Autodesk Inventor part; units mm, degrees
(part 3 of 3)
sketch "스케치33" plane through (0, 0, 2) normal (0, 0, 1) x (1, 0, 0)
  circle A0 centre (-11.9, -60) radius 1.35 projected
  line L0 (-6.96, -60.06) -> (-6.96, -57.94) projected
  arc A1 (-4.76, -57.94) -> (-6.96, -57.94) centre (-5.86, -57.94) ccw projected
  line L1 (-4.76, -57.94) -> (4.96, -57.94) projected
  arc A2 (7.16, -57.94) -> (4.96, -57.94) centre (6.06, -57.94) ccw projected
  line L2 (7.16, -57.94) -> (7.16, -60.06) projected
  arc A3 (4.96, -60.06) -> (7.16, -60.06) centre (6.06, -60.06) ccw projected
  line L3 (4.96, -60.06) -> (-4.76, -60.06) projected
  arc A4 (-6.96, -60.06) -> (-4.76, -60.06) centre (-5.86, -60.06) ccw projected
  circle A5 centre (12.1, -60) radius 1.35 projected
  line L4 (-14.9, -62) -> (15.1, -62) projected
  line L5 (15.1, -62) -> (15.1, -54.5339) projected
  arc A6 (15.1, -54.5339) -> (14.9713, -53.4701) centre (10.639, -54.5339) ccw projected
  line L6 (14.9713, -53.4701) -> (6.3746, -18.4593) projected
  arc A7 (6.3746, -18.4593) -> (-6.1746, -18.4593) centre (0.1, -20) ccw projected
  line L7 (-6.1746, -18.4593) -> (-14.7713, -53.4701) projected
  arc A8 (-14.7713, -53.4701) -> (-14.9, -54.5339) centre (-10.439, -54.5339) ccw projected
  line L8 (-14.9, -54.5339) -> (-14.9, -62) projected
  line L9 (-8.6217, -47.1327) -> (-4.5428, -30.5211) projected
  arc A9 (-0.3945, -27.4837) -> (-4.5428, -30.5211) centre (-0.6582, -31.475) ccw projected
  arc A10 (-0.3945, -27.4837) -> (0.5945, -27.4837) centre (0.1, -20) ccw projected
  arc A11 (4.7428, -30.5211) -> (0.5945, -27.4837) centre (0.8582, -31.475) ccw projected
  line L10 (4.7428, -30.5211) -> (8.8217, -47.1327) projected
  arc A12 (5.616, -52.0285) -> (8.8217, -47.1327) centre (4.9371, -48.0865) ccw projected
  arc A13 (-5.416, -52.0285) -> (5.616, -52.0285) centre (0.1, -20) ccw projected
  arc A14 (-8.6217, -47.1327) -> (-5.416, -52.0285) centre (-4.7371, -48.0865) ccw projected
  circle A15 centre (0.1, -20) radius 4 projected
  circle A16 centre (0.1, -20) radius 4 projected
  line L11 (-15.822, -62) -> (16.178, -62) projected
  line L12 (16.178, -62) -> (16.178, -54.5339) projected
  arc A17 (16.178, -54.5339) -> (16.0205, -53.2317) centre (10.717, -54.5339) ccw projected
  line L13 (16.0205, -53.2317) -> (7.4238, -18.2208) projected
  arc A18 (7.4238, -18.2208) -> (-7.0677, -18.2208) centre (0.178, -20) ccw projected
  line L14 (-7.0677, -18.2208) -> (-15.6644, -53.2317) projected
  arc A19 (-15.6644, -53.2317) -> (-15.822, -54.5339) centre (-10.361, -54.5339) ccw projected
  line L15 (-15.822, -54.5339) -> (-15.822, -62) projected
  circle A20 centre (11.1, -45.3) radius 1.35 projected
  line L16 (8.16, -44.34) -> (8.16, -46.26) projected
  arc A21 (7.06, -47.36) -> (8.16, -46.26) centre (8.16, -47.36) ccw projected
  line L17 (7.06, -47.36) -> (-6.86, -47.36) projected
  arc A22 (-7.96, -46.26) -> (-6.86, -47.36) centre (-7.96, -47.36) ccw projected
  line L18 (-7.96, -46.26) -> (-7.96, -44.34) projected
  arc A23 (-6.86, -43.24) -> (-7.96, -44.34) centre (-7.96, -43.24) ccw projected
  line L19 (-6.86, -43.24) -> (7.06, -43.24) projected
  arc A24 (8.16, -44.34) -> (7.06, -43.24) centre (8.16, -43.24) ccw projected
  circle A25 centre (-10.9, -45.3) radius 1.35 projected
  arc A26 (-4.9649, -40.6273) -> (5.1649, -40.6273) centre (0.1, -20) ccw projected
  arc A27 (-6.4303, -38.208) -> (-4.9649, -40.6273) centre (-4.488, -38.685) ccw projected
  line L20 (-6.4303, -38.208) -> (-4.5428, -30.5211) projected
  arc A28 (-0.3945, -27.4837) -> (-4.5428, -30.5211) centre (-0.6582, -31.475) ccw projected
  arc A29 (-0.3945, -27.4837) -> (0.5945, -27.4837) centre (0.1, -20) ccw projected
  arc A30 (4.7428, -30.5211) -> (0.5945, -27.4837) centre (0.8582, -31.475) ccw projected
  line L21 (4.7428, -30.5211) -> (6.6303, -38.208) projected
  arc A31 (5.1649, -40.6273) -> (6.6303, -38.208) centre (4.688, -38.685) ccw projected
  point P0 (0, 0)
extrude "돌출33" cut sketch "스케치33" against normal blind 2 contours A0 | L0 A1 L1 A2 L2 A3 L3 A4 | A5
sketch "스케치34" plane through (0, 0, 2) normal (0, 0, 1) x (1, 0, 0)
  circle A0 centre (12.1, -60) radius 1.35 projected
  circle A1 centre (-11.9, -60) radius 1.35 projected
  arc A2 (7.16, -57.94) -> (4.96, -57.94) centre (6.06, -57.94) ccw projected
  line L0 (7.16, -57.94) -> (7.16, -60.06) projected
  arc A3 (4.96, -60.06) -> (7.16, -60.06) centre (6.06, -60.06) ccw projected
  line L1 (4.96, -60.06) -> (-4.76, -60.06) projected
  arc A4 (-6.96, -60.06) -> (-4.76, -60.06) centre (-5.86, -60.06) ccw projected
  line L2 (-6.96, -60.06) -> (-6.96, -57.94) projected
  arc A5 (-4.76, -57.94) -> (-6.96, -57.94) centre (-5.86, -57.94) ccw projected
  line L3 (-4.76, -57.94) -> (4.96, -57.94) projected
  circle A6 centre (0.1, -20) radius 4 projected
  line L4 (-15.822, -62) -> (16.178, -62) projected
  line L5 (16.178, -62) -> (16.178, -54.5339) projected
  arc A7 (16.178, -54.5339) -> (16.0205, -53.2317) centre (10.717, -54.5339) ccw projected
  line L6 (16.0205, -53.2317) -> (7.4238, -18.2208) projected
  arc A8 (7.4238, -18.2208) -> (-7.0677, -18.2208) centre (0.178, -20) ccw projected
  line L7 (-7.0677, -18.2208) -> (-15.6644, -53.2317) projected
  arc A9 (-15.6644, -53.2317) -> (-15.822, -54.5339) centre (-10.361, -54.5339) ccw projected
  line L8 (-15.822, -54.5339) -> (-15.822, -62) projected
  circle A10 centre (11.1, -45.3) radius 1.35 projected
  line L9 (8.16, -44.34) -> (8.16, -46.26) projected
  arc A11 (7.06, -47.36) -> (8.16, -46.26) centre (8.16, -47.36) ccw projected
  line L10 (7.06, -47.36) -> (-6.86, -47.36) projected
  arc A12 (-7.96, -46.26) -> (-6.86, -47.36) centre (-7.96, -47.36) ccw projected
  line L11 (-7.96, -46.26) -> (-7.96, -44.34) projected
  arc A13 (-6.86, -43.24) -> (-7.96, -44.34) centre (-7.96, -43.24) ccw projected
  line L12 (-6.86, -43.24) -> (7.06, -43.24) projected
  arc A14 (8.16, -44.34) -> (7.06, -43.24) centre (8.16, -43.24) ccw projected
  circle A15 centre (-10.9, -45.3) radius 1.35 projected
  arc A16 (-4.9649, -40.6273) -> (5.1649, -40.6273) centre (0.1, -20) ccw projected
  arc A17 (-6.4303, -38.208) -> (-4.9649, -40.6273) centre (-4.488, -38.685) ccw projected
  line L13 (-6.4303, -38.208) -> (-4.5428, -30.5211) projected
  arc A18 (-0.3945, -27.4837) -> (-4.5428, -30.5211) centre (-0.6582, -31.475) ccw projected
  arc A19 (-0.3945, -27.4837) -> (0.5945, -27.4837) centre (0.1, -20) ccw projected
  arc A20 (4.7428, -30.5211) -> (0.5945, -27.4837) centre (0.8582, -31.475) ccw projected
  line L14 (4.7428, -30.5211) -> (6.6303, -38.208) projected
  arc A21 (5.1649, -40.6273) -> (6.6303, -38.208) centre (4.688, -38.685) ccw projected
  circle A22 centre (-11.9, -60) radius 1.35 projected
  line L15 (-6.96, -60.06) -> (-6.96, -57.94) projected
  arc A23 (-4.76, -57.94) -> (-6.96, -57.94) centre (-5.86, -57.94) ccw projected
  line L16 (-4.76, -57.94) -> (4.96, -57.94) projected
  arc A24 (7.16, -57.94) -> (4.96, -57.94) centre (6.06, -57.94) ccw projected
  line L17 (7.16, -57.94) -> (7.16, -60.06) projected
  arc A25 (4.96, -60.06) -> (7.16, -60.06) centre (6.06, -60.06) ccw projected
  line L18 (4.96, -60.06) -> (-4.76, -60.06) projected
  arc A26 (-6.96, -60.06) -> (-4.76, -60.06) centre (-5.86, -60.06) ccw projected
  circle A27 centre (12.1, -60) radius 1.35 projected
  line L19 (-14.9, -62) -> (15.1, -62) projected
  line L20 (15.1, -62) -> (15.1, -54.5339) projected
  arc A28 (15.1, -54.5339) -> (14.9713, -53.4701) centre (10.639, -54.5339) ccw projected
  line L21 (14.9713, -53.4701) -> (6.3746, -18.4593) projected
  arc A29 (6.3746, -18.4593) -> (-6.1746, -18.4593) centre (0.1, -20) ccw projected
  line L22 (-6.1746, -18.4593) -> (-14.7713, -53.4701) projected
  arc A30 (-14.7713, -53.4701) -> (-14.9, -54.5339) centre (-10.439, -54.5339) ccw projected
  line L23 (-14.9, -54.5339) -> (-14.9, -62) projected
  line L24 (-8.6217, -47.1327) -> (-4.5428, -30.5211) projected
  arc A31 (-0.3945, -27.4837) -> (-4.5428, -30.5211) centre (-0.6582, -31.475) ccw projected
  arc A32 (-0.3945, -27.4837) -> (0.5945, -27.4837) centre (0.1, -20) ccw projected
  arc A33 (4.7428, -30.5211) -> (0.5945, -27.4837) centre (0.8582, -31.475) ccw projected
  line L25 (4.7428, -30.5211) -> (8.8217, -47.1327) projected
  arc A34 (5.616, -52.0285) -> (8.8217, -47.1327) centre (4.9371, -48.0865) ccw projected
  arc A35 (-5.416, -52.0285) -> (5.616, -52.0285) centre (0.1, -20) ccw projected
  arc A36 (-8.6217, -47.1327) -> (-5.416, -52.0285) centre (-4.7371, -48.0865) ccw projected
  circle A37 centre (0.1, -20) radius 4 projected
  point P0 (0, 0)
extrude "돌출34" cut sketch "스케치34" against normal blind 2 contours L8 A9 L7 A8 L6 A7 L5 L4 L20 A28 L21 A29 L22 A30 L23
sketch "스케치35" plane through (0, 0, 2) normal (0, 0, 1) x (1, 0, 0)
  arc A0 (-4.9649, -40.6273) -> (5.1649, -40.6273) centre (0.1, -20) ccw projected
  arc A1 (-6.4303, -38.208) -> (-4.9649, -40.6273) centre (-4.488, -38.685) ccw projected
  line L0 (-6.4303, -38.208) -> (-4.5428, -30.5211) projected
  arc A2 (-0.3945, -27.4837) -> (-4.5428, -30.5211) centre (-0.6582, -31.475) ccw projected
  arc A3 (-0.3945, -27.4837) -> (0.5945, -27.4837) centre (0.1, -20) ccw projected
  arc A4 (4.7428, -30.5211) -> (0.5945, -27.4837) centre (0.8582, -31.475) ccw projected
  line L1 (4.7428, -30.5211) -> (6.6303, -38.208) projected
  arc A5 (5.1649, -40.6273) -> (6.6303, -38.208) centre (4.688, -38.685) ccw projected
  circle A6 centre (-10.9, -45.3) radius 1.35 projected
  line L2 (8.16, -44.34) -> (8.16, -46.26) projected
  arc A7 (7.06, -47.36) -> (8.16, -46.26) centre (8.16, -47.36) ccw projected
  line L3 (7.06, -47.36) -> (-6.86, -47.36) projected
  arc A8 (-7.96, -46.26) -> (-6.86, -47.36) centre (-7.96, -47.36) ccw projected
  line L4 (-7.96, -46.26) -> (-7.96, -44.34) projected
  arc A9 (-6.86, -43.24) -> (-7.96, -44.34) centre (-7.96, -43.24) ccw projected
  line L5 (-6.86, -43.24) -> (7.06, -43.24) projected
  arc A10 (8.16, -44.34) -> (7.06, -43.24) centre (8.16, -43.24) ccw projected
  circle A11 centre (11.1, -45.3) radius 1.35 projected
  line L6 (15.1, -62) -> (15.1, -54.5339) projected
  arc A12 (15.1, -54.5339) -> (14.9713, -53.4701) centre (10.639, -54.5339) ccw projected
  line L7 (14.9713, -53.4701) -> (6.3746, -18.4593) projected
  arc A13 (6.3746, -18.4593) -> (-6.1746, -18.4593) centre (0.1, -20) ccw projected
  line L8 (-6.1746, -18.4593) -> (-14.7713, -53.4701) projected
  arc A14 (-14.7713, -53.4701) -> (-14.9, -54.5339) centre (-10.439, -54.5339) ccw projected
  line L9 (-14.9, -54.5339) -> (-14.9, -62) projected
  line L10 (-14.9, -62) -> (15.1, -62) projected
  circle A15 centre (0.1, -20) radius 4 projected
  arc A16 (7.16, -57.94) -> (4.96, -57.94) centre (6.06, -57.94) ccw projected
  line L11 (7.16, -57.94) -> (7.16, -60.06) projected
  arc A17 (4.96, -60.06) -> (7.16, -60.06) centre (6.06, -60.06) ccw projected
  line L12 (4.96, -60.06) -> (-4.76, -60.06) projected
  arc A18 (-6.96, -60.06) -> (-4.76, -60.06) centre (-5.86, -60.06) ccw projected
  line L13 (-6.96, -60.06) -> (-6.96, -57.94) projected
  arc A19 (-4.76, -57.94) -> (-6.96, -57.94) centre (-5.86, -57.94) ccw projected
  line L14 (-4.76, -57.94) -> (4.96, -57.94) projected
  circle A20 centre (-11.9, -60) radius 1.35 projected
  circle A21 centre (12.1, -60) radius 1.35 projected
  line L15 (16.1, -54.5339) -> (16.1, -63)
  line L16 (16.1, -63) -> (-15.9, -63)
  line L17 (-15.9, -63) -> (-15.9, -54.5339)
  arc A22 (-15.7425, -53.2317) -> (-15.9, -54.5339) centre (-10.439, -54.5339) ccw
  line L18 (-15.7425, -53.2317) -> (-7.1458, -18.2208)
  arc A23 (7.3458, -18.2208) -> (-7.1458, -18.2208) centre (0.1, -20) ccw
  line L19 (7.3458, -18.2208) -> (15.9425, -53.2317)
  arc A24 (16.1, -54.5339) -> (15.9425, -53.2317) centre (10.639, -54.5339) ccw
  line L20 (16.1, -63) -> (-15.9, -63)
  line L21 (-15.9, -63) -> (-15.9, -62)
  line L22 (-15.9, -62) -> (16.1, -62)
  line L23 (16.1, -62) -> (16.1, -63)
  point P0 (0, 0)
  dimension "d134" = 1
  constraints: 18 end point, 6 point on circle, 3 centre point, 2 parallel, 1 horizontal, 1 perpendicular, 7 other
  measures "d134" distance between parallel lines of L6 L15
extrude "돌출35" add sketch "스케치35" against normal blind 2 contours L6 A12 L7 A13 L8 A14 L9 L22 L17 A22 L18 A23 L19 A24 L15
sketch "스케치36" plane through (0, 0, 0) normal (0, 0, -1) x (-1, 0, 0)
  line L0 (-16.1, -62) -> (15.9, -62) projected
  line L1 (15.9, -62) -> (15.9, -54.5339) projected
  arc A0 (15.9, -54.5339) -> (15.7425, -53.2317) centre (10.439, -54.5339) ccw projected
  line L2 (15.7425, -53.2317) -> (7.1458, -18.2208) projected
  arc A1 (7.1458, -18.2208) -> (-7.3458, -18.2208) centre (-0.1, -20) ccw projected
  line L3 (-7.3458, -18.2208) -> (-15.9425, -53.2317) projected
  arc A2 (-15.9425, -53.2317) -> (-16.1, -54.5339) centre (-10.639, -54.5339) ccw projected
  line L4 (-16.1, -54.5339) -> (-16.1, -62) projected
  circle A3 centre (-12.1, -60) radius 1.35 projected
  circle A4 centre (11.9, -60) radius 1.35 projected
  arc A5 (-4.96, -57.94) -> (-7.16, -57.94) centre (-6.06, -57.94) ccw projected
  line L5 (-4.96, -57.94) -> (4.76, -57.94) projected
  arc A6 (6.96, -57.94) -> (4.76, -57.94) centre (5.86, -57.94) ccw projected
  line L6 (6.96, -57.94) -> (6.96, -60.06) projected
  arc A7 (4.76, -60.06) -> (6.96, -60.06) centre (5.86, -60.06) ccw projected
  line L7 (4.76, -60.06) -> (-4.96, -60.06) projected
  arc A8 (-7.16, -60.06) -> (-4.96, -60.06) centre (-6.06, -60.06) ccw projected
  line L8 (-7.16, -60.06) -> (-7.16, -57.94) projected
  arc A9 (-5.1649, -40.6273) -> (4.9649, -40.6273) centre (-0.1, -20) ccw projected
  arc A10 (-6.6303, -38.208) -> (-5.1649, -40.6273) centre (-4.688, -38.685) ccw projected
  line L9 (-6.6303, -38.208) -> (-4.7428, -30.5211) projected
  arc A11 (-0.5945, -27.4837) -> (-4.7428, -30.5211) centre (-0.8582, -31.475) ccw projected
  arc A12 (-0.5945, -27.4837) -> (0.3945, -27.4837) centre (-0.1, -20) ccw projected
  arc A13 (4.5428, -30.5211) -> (0.3945, -27.4837) centre (0.6582, -31.475) ccw projected
  line L10 (4.5428, -30.5211) -> (6.4303, -38.208) projected
  arc A14 (4.9649, -40.6273) -> (6.4303, -38.208) centre (4.488, -38.685) ccw projected
  circle A15 centre (10.9, -45.3) radius 1.35 projected
  line L11 (-8.16, -46.26) -> (-8.16, -44.34) projected
  arc A16 (-7.06, -43.24) -> (-8.16, -44.34) centre (-8.16, -43.24) ccw projected
  line L12 (-7.06, -43.24) -> (6.86, -43.24) projected
  arc A17 (7.96, -44.34) -> (6.86, -43.24) centre (7.96, -43.24) ccw projected
  line L13 (7.96, -44.34) -> (7.96, -46.26) projected
  arc A18 (6.86, -47.36) -> (7.96, -46.26) centre (7.96, -47.36) ccw projected
  line L14 (6.86, -47.36) -> (-7.06, -47.36) projected
  arc A19 (-8.16, -46.26) -> (-7.06, -47.36) centre (-8.16, -47.36) ccw projected
  circle A20 centre (-11.1, -45.3) radius 1.35 projected
  circle A21 centre (-0.1, -20) radius 4 projected
  point P0 (0, 0)
extrude "돌출36" add sketch "스케치36" against normal blind 2 contours L5 A6 L6 A7 L7 A8 L8 A5
sketch "스케치37" plane through (0, 0, 2) normal (0, 0, 1) x (1, 0, 0)
  arc A0 (-5.86, -57.94) -> (-6.96, -59.04) centre (-6.96, -57.94) ccw projected
  line L0 (-5.86, -57.94) -> (6.06, -57.94) projected
  arc A1 (7.16, -59.04) -> (6.06, -57.94) centre (7.16, -57.94) ccw projected
  line L1 (7.16, -59.04) -> (7.16, -62) projected
  line L2 (7.16, -62) -> (15.1, -62) projected
  line L3 (15.1, -62) -> (15.1, -54.5339) projected
  arc A2 (15.1, -54.5339) -> (14.9713, -53.4701) centre (10.639, -54.5339) ccw projected
  line L4 (14.9713, -53.4701) -> (6.3746, -18.4593) projected
  arc A3 (6.3746, -18.4593) -> (-6.1746, -18.4593) centre (0.1, -20) ccw projected
  line L5 (-6.1746, -18.4593) -> (-14.7713, -53.4701) projected
  arc A4 (-14.7713, -53.4701) -> (-14.9, -54.5339) centre (-10.439, -54.5339) ccw projected
  line L6 (-14.9, -54.5339) -> (-14.9, -62) projected
  line L7 (-14.9, -62) -> (-6.96, -62) projected
  line L8 (-6.96, -62) -> (-6.96, -59.04) projected
  circle A5 centre (-11.9, -60) radius 1.35 projected
  circle A6 centre (12.1, -60) radius 1.35 projected
  line L9 (-8.6217, -47.1327) -> (-4.5428, -30.5211) projected
  arc A7 (-0.3945, -27.4837) -> (-4.5428, -30.5211) centre (-0.6582, -31.475) ccw projected
  arc A8 (-0.3945, -27.4837) -> (0.5945, -27.4837) centre (0.1, -20) ccw projected
  arc A9 (4.7428, -30.5211) -> (0.5945, -27.4837) centre (0.8582, -31.475) ccw projected
  line L10 (4.7428, -30.5211) -> (8.8217, -47.1327) projected
  arc A10 (5.616, -52.0285) -> (8.8217, -47.1327) centre (4.9371, -48.0865) ccw projected
  arc A11 (-5.416, -52.0285) -> (5.616, -52.0285) centre (0.1, -20) ccw projected
  arc A12 (-8.6217, -47.1327) -> (-5.416, -52.0285) centre (-4.7371, -48.0865) ccw projected
  circle A13 centre (0.1, -20) radius 4 projected
  arc A14 (-4.9649, -40.6273) -> (5.1649, -40.6273) centre (0.1, -20) ccw projected
  arc A15 (-6.4303, -38.208) -> (-4.9649, -40.6273) centre (-4.488, -38.685) ccw projected
  line L11 (-6.4303, -38.208) -> (-4.5428, -30.5211) projected
  arc A16 (-0.3945, -27.4837) -> (-4.5428, -30.5211) centre (-0.6582, -31.475) ccw projected
  arc A17 (-0.3945, -27.4837) -> (0.5945, -27.4837) centre (0.1, -20) ccw projected
  arc A18 (4.7428, -30.5211) -> (0.5945, -27.4837) centre (0.8582, -31.475) ccw projected
  line L12 (4.7428, -30.5211) -> (6.6303, -38.208) projected
  arc A19 (5.1649, -40.6273) -> (6.6303, -38.208) centre (4.688, -38.685) ccw projected
  circle A20 centre (-10.9, -45.3) radius 1.35 projected
  line L13 (8.16, -44.34) -> (8.16, -46.26) projected
  arc A21 (7.06, -47.36) -> (8.16, -46.26) centre (8.16, -47.36) ccw projected
  line L14 (7.06, -47.36) -> (-6.86, -47.36) projected
  arc A22 (-7.96, -46.26) -> (-6.86, -47.36) centre (-7.96, -47.36) ccw projected
  line L15 (-7.96, -46.26) -> (-7.96, -44.34) projected
  arc A23 (-6.86, -43.24) -> (-7.96, -44.34) centre (-7.96, -43.24) ccw projected
  line L16 (-6.86, -43.24) -> (7.06, -43.24) projected
  arc A24 (8.16, -44.34) -> (7.06, -43.24) centre (8.16, -43.24) ccw projected
  circle A25 centre (11.1, -45.3) radius 1.35 projected
  line L17 (-15.9, -62) -> (16.1, -62) projected
  line L18 (16.1, -62) -> (16.1, -54.5339) projected
  arc A26 (16.1, -54.5339) -> (15.9425, -53.2317) centre (10.639, -54.5339) ccw projected
  line L19 (15.9425, -53.2317) -> (7.3458, -18.2208) projected
  arc A27 (7.3458, -18.2208) -> (-7.1458, -18.2208) centre (0.1, -20) ccw projected
  line L20 (-7.1458, -18.2208) -> (-15.7425, -53.2317) projected
  arc A28 (-15.7425, -53.2317) -> (-15.9, -54.5339) centre (-10.439, -54.5339) ccw projected
  line L21 (-15.9, -54.5339) -> (-15.9, -62) projected
  circle A29 centre (0.1, -20) radius 4 projected
  circle A30 centre (-11.9, -60) radius 1.35 projected
  circle A31 centre (12.1, -60) radius 1.35 projected
  point P0 (0, 0)
extrude "돌출37" cut sketch "스케치37" against normal through all contours L0 A1 L1 L17 L8 A0
sketch "스케치38" plane through (0, 0, 2) normal (0, 0, 1) x (1, 0, 0)
  circle A0 centre (12.1, -60) radius 1.35 projected
  circle A1 centre (-11.9, -60) radius 1.35 projected
  circle A2 centre (0.1, -20) radius 4 projected
  line L0 (-6.96, -62) -> (-6.96, -59.04) projected
  arc A3 (-5.86, -57.94) -> (-6.96, -59.04) centre (-6.96, -57.94) ccw projected
  line L1 (-5.86, -57.94) -> (6.06, -57.94) projected
  arc A4 (7.16, -59.04) -> (6.06, -57.94) centre (7.16, -57.94) ccw projected
  line L2 (7.16, -59.04) -> (7.16, -62) projected
  line L3 (7.16, -62) -> (16.1, -62) projected
  line L4 (16.1, -62) -> (16.1, -54.5339) projected
  arc A5 (16.1, -54.5339) -> (15.9425, -53.2317) centre (10.639, -54.5339) ccw projected
  line L5 (15.9425, -53.2317) -> (7.3458, -18.2208) projected
  arc A6 (7.3458, -18.2208) -> (-7.1458, -18.2208) centre (0.1, -20) ccw projected
  line L6 (-7.1458, -18.2208) -> (-15.7425, -53.2317) projected
  arc A7 (-15.7425, -53.2317) -> (-15.9, -54.5339) centre (-10.439, -54.5339) ccw projected
  line L7 (-15.9, -54.5339) -> (-15.9, -62) projected
  line L8 (-15.9, -62) -> (-6.96, -62) projected
  circle A8 centre (11.1, -45.3) radius 1.35 projected
  line L9 (8.16, -44.34) -> (8.16, -46.26) projected
  arc A9 (7.06, -47.36) -> (8.16, -46.26) centre (8.16, -47.36) ccw projected
  line L10 (7.06, -47.36) -> (-6.86, -47.36) projected
  arc A10 (-7.96, -46.26) -> (-6.86, -47.36) centre (-7.96, -47.36) ccw projected
  line L11 (-7.96, -46.26) -> (-7.96, -44.34) projected
  arc A11 (-6.86, -43.24) -> (-7.96, -44.34) centre (-7.96, -43.24) ccw projected
  line L12 (-6.86, -43.24) -> (7.06, -43.24) projected
  arc A12 (8.16, -44.34) -> (7.06, -43.24) centre (8.16, -43.24) ccw projected
  circle A13 centre (-10.9, -45.3) radius 1.35 projected
  arc A14 (-4.9649, -40.6273) -> (5.1649, -40.6273) centre (0.1, -20) ccw projected
  arc A15 (-6.4303, -38.208) -> (-4.9649, -40.6273) centre (-4.488, -38.685) ccw projected
  line L13 (-6.4303, -38.208) -> (-4.5428, -30.5211) projected
  arc A16 (-0.3945, -27.4837) -> (-4.5428, -30.5211) centre (-0.6582, -31.475) ccw projected
  arc A17 (-0.3945, -27.4837) -> (0.5945, -27.4837) centre (0.1, -20) ccw projected
  arc A18 (4.7428, -30.5211) -> (0.5945, -27.4837) centre (0.8582, -31.475) ccw projected
  line L14 (4.7428, -30.5211) -> (6.6303, -38.208) projected
  arc A19 (5.1649, -40.6273) -> (6.6303, -38.208) centre (4.688, -38.685) ccw projected
  circle A20 centre (0.1, -20) radius 2
  point P0 (0, 0)
  dimension "d141" = 4
  constraints: 1 centre point, 1 coincident
  measures "d141" diameter of A20
extrude "돌출38" add sketch "스케치38" against normal up to surface (2 mm away) contours A2
sketch "스케치39" plane through (0, 0, 0) normal (0, 0, -1) x (-1, 0, 0)
  circle A0 centre (-0.1, -20) radius 2 projected
  circle A1 centre (-11.1, -45.3) radius 1.35 projected
  line L0 (-8.16, -46.26) -> (-8.16, -44.34) projected
  arc A2 (-7.06, -43.24) -> (-8.16, -44.34) centre (-8.16, -43.24) ccw projected
  line L1 (-7.06, -43.24) -> (6.86, -43.24) projected
  arc A3 (7.96, -44.34) -> (6.86, -43.24) centre (7.96, -43.24) ccw projected
  line L2 (7.96, -44.34) -> (7.96, -46.26) projected
  arc A4 (6.86, -47.36) -> (7.96, -46.26) centre (7.96, -47.36) ccw projected
  line L3 (6.86, -47.36) -> (-7.06, -47.36) projected
  arc A5 (-8.16, -46.26) -> (-7.06, -47.36) centre (-8.16, -47.36) ccw projected
  circle A6 centre (10.9, -45.3) radius 1.35 projected
  arc A7 (-5.1649, -40.6273) -> (4.9649, -40.6273) centre (-0.1, -20) ccw projected
  arc A8 (-6.6303, -38.208) -> (-5.1649, -40.6273) centre (-4.688, -38.685) ccw projected
  line L4 (-6.6303, -38.208) -> (-4.7428, -30.5211) projected
  arc A9 (-0.5945, -27.4837) -> (-4.7428, -30.5211) centre (-0.8582, -31.475) ccw projected
  arc A10 (-0.5945, -27.4837) -> (0.3945, -27.4837) centre (-0.1, -20) ccw projected
  arc A11 (4.5428, -30.5211) -> (0.3945, -27.4837) centre (0.6582, -31.475) ccw projected
  line L5 (4.5428, -30.5211) -> (6.4303, -38.208) projected
  arc A12 (4.9649, -40.6273) -> (6.4303, -38.208) centre (4.488, -38.685) ccw projected
  circle A13 centre (11.9, -60) radius 1.35 projected
  circle A14 centre (-12.1, -60) radius 1.35 projected
  line L6 (-7.16, -62) -> (-7.16, -59.04) projected
  arc A15 (-6.06, -57.94) -> (-7.16, -59.04) centre (-7.16, -57.94) ccw projected
  line L7 (-6.06, -57.94) -> (5.86, -57.94) projected
  arc A16 (6.96, -59.04) -> (5.86, -57.94) centre (6.96, -57.94) ccw projected
  line L8 (6.96, -59.04) -> (6.96, -62) projected
  line L9 (6.96, -62) -> (15.9, -62) projected
  line L10 (15.9, -62) -> (15.9, -54.5339) projected
  arc A17 (15.9, -54.5339) -> (15.7425, -53.2317) centre (10.439, -54.5339) ccw projected
  line L11 (15.7425, -53.2317) -> (7.1458, -18.2208) projected
  arc A18 (7.1458, -18.2208) -> (-7.3458, -18.2208) centre (-0.1, -20) ccw projected
  line L12 (-7.3458, -18.2208) -> (-15.9425, -53.2317) projected
  arc A19 (-15.9425, -53.2317) -> (-16.1, -54.5339) centre (-10.639, -54.5339) ccw projected
  line L13 (-16.1, -54.5339) -> (-16.1, -62) projected
  line L14 (-16.1, -62) -> (-7.16, -62) projected
  point P0 (0, 0)
extrude "돌출39" add sketch "스케치39" along normal blind 1
sketch "스케치40" plane through (0, 0, -1) normal (0, 0, -1) x (-1, 0, 0)
  line L0 (6.96, -62) -> (15.9, -62) projected
  line L1 (15.9, -62) -> (15.9, -54.5339) projected
  arc A0 (15.9, -54.5339) -> (15.7425, -53.2317) centre (10.439, -54.5339) ccw projected
  line L2 (15.7425, -53.2317) -> (7.1458, -18.2208) projected
  arc A1 (7.1458, -18.2208) -> (-7.3458, -18.2208) centre (-0.1, -20) ccw projected
  line L3 (-7.3458, -18.2208) -> (-15.9425, -53.2317) projected
  arc A2 (-15.9425, -53.2317) -> (-16.1, -54.5339) centre (-10.639, -54.5339) ccw projected
  line L4 (-16.1, -54.5339) -> (-16.1, -62) projected
  line L5 (-16.1, -62) -> (-7.16, -62) projected
  line L6 (-7.16, -62) -> (-7.16, -59.04) projected
  arc A3 (-6.06, -57.94) -> (-7.16, -59.04) centre (-7.16, -57.94) ccw projected
  line L7 (-6.06, -57.94) -> (5.86, -57.94) projected
  arc A4 (6.96, -59.04) -> (5.86, -57.94) centre (6.96, -57.94) ccw projected
  line L8 (6.96, -59.04) -> (6.96, -62) projected
  circle A5 centre (11.9, -60) radius 1.35 projected
  circle A6 centre (-12.1, -60) radius 1.35 projected
  line L9 (-6.6303, -38.208) -> (-4.7428, -30.5211) projected
  arc A7 (-0.5945, -27.4837) -> (-4.7428, -30.5211) centre (-0.8582, -31.475) ccw projected
  arc A8 (-0.5945, -27.4837) -> (0.3945, -27.4837) centre (-0.1, -20) ccw projected
  arc A9 (4.5428, -30.5211) -> (0.3945, -27.4837) centre (0.6582, -31.475) ccw projected
  line L10 (4.5428, -30.5211) -> (6.4303, -38.208) projected
  arc A10 (4.9649, -40.6273) -> (6.4303, -38.208) centre (4.488, -38.685) ccw projected
  arc A11 (-5.1649, -40.6273) -> (4.9649, -40.6273) centre (-0.1, -20) ccw projected
  arc A12 (-6.6303, -38.208) -> (-5.1649, -40.6273) centre (-4.688, -38.685) ccw projected
  circle A13 centre (10.9, -45.3) radius 1.35 projected
  line L11 (6.86, -47.36) -> (-7.06, -47.36) projected
  arc A14 (-8.16, -46.26) -> (-7.06, -47.36) centre (-8.16, -47.36) ccw projected
  line L12 (-8.16, -46.26) -> (-8.16, -44.34) projected
  arc A15 (-7.06, -43.24) -> (-8.16, -44.34) centre (-8.16, -43.24) ccw projected
  line L13 (-7.06, -43.24) -> (6.86, -43.24) projected
  arc A16 (7.96, -44.34) -> (6.86, -43.24) centre (7.96, -43.24) ccw projected
  line L14 (7.96, -44.34) -> (7.96, -46.26) projected
  arc A17 (6.86, -47.36) -> (7.96, -46.26) centre (7.96, -47.36) ccw projected
  circle A18 centre (-11.1, -45.3) radius 1.35 projected
  circle A19 centre (-0.1, -20) radius 2 projected
  circle A20 centre (-0.1, -20) radius 4
  point P0 (0, 0)
  dimension "d146" = 8
  constraints: 1 centre point, 1 coincident
  measures "d146" diameter of A20
extrude "돌출40" cut sketch "스케치40" against normal through all contours A19 | A20
